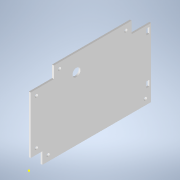
# Autodesk Inventor part: Steckerplatte_hint
Saved by Autodesk Inventor 2022 (Build 260153000, 153)
## iProperties
Created: 2022-02-01
Part Number: Steckerplatte_hint
Material: Generic
Document SubType Name: Modeling
Designer: Fabijansven
Density: 1 g/cm^3
Appearance: Default
Author: Fabijansven
Autodesk Inventor part; units mm, degrees
ref_plane "YZ Plane" through (0, 0, 0) normal (1, 0, 0) x (0, 1, 0)
ref_plane "XZ Plane" through (0, 0, 0) normal (0, 1, 0) x (-1, 0, 0)
ref_plane "XY Plane" through (0, 0, 0) normal (0, 0, 1) x (1, 0, 0)
sketch "Sketch1" plane through (0, 0, 0) normal (1, 0, 0) x (0, 1, 0)
  line L0 (0, 0) -> (140, 0)
  line L1 (140, 0) -> (140, -210)
  line L2 (140, -210) -> (0, -210)
  line L3 (0, -210) -> (0, 0)
  dimension "d0" = 210
  dimension "d1" = 140
  constraints: 8 end point, 2 parallel, 1 horizontal, 1 perpendicular
  measures "d0" distance of L0.end L1.end
  measures "d1" distance of L1.end L2.end
extrude "Extrusion1" add sketch "Sketch1" along normal blind 3
sketch "Sketch2" plane through (0, 0, 0) normal (-1, 0, 0) x (0, 0, 1)
  line L0 (0, 0) -> (-20.5, 0)
  line L1 (-20.5, 0) -> (-20.5, 20.5)
  line L2 (-20.5, 20.5) -> (0, 20.5)
  line L3 (0, 20.5) -> (0, 0)
  line L4 (-210, 140) -> (0, 140) projected
  line L5 (0, 140) -> (-40.5, 140)
  line L6 (-40.5, 140) -> (-40.5, 119.5)
  line L7 (-40.5, 119.5) -> (0, 119.5)
  line L8 (0, 119.5) -> (0, 140)
  line L9 (-210, 140) -> (-176, 140)
  line L10 (-176, 140) -> (-176, 119.5)
  line L11 (-176, 119.5) -> (-210, 119.5)
  line L12 (-210, 119.5) -> (-210, 140)
  point P0 (-176, 140)
  dimension "d4" = 20.5
  dimension "d5" = 20.5
  dimension "d6" = 40.5
  dimension "d7" = 20.5
  dimension "d8" = 34
  constraints: 24 end point, 6 parallel, 3 horizontal, 3 perpendicular, 1 point on line
  measures "d4" distance of L0.end L1.end
  measures "d5" distance of L5.end L6.end
  measures "d6" distance between parallel lines of L8 L6
  measures "d7" distance of L1.end L2.end
  measures "d8" distance between parallel lines of L12 L10
extrude "Extrusion2" cut sketch "Sketch2" against normal blind 3
sketch "Sketch3" plane through (0, 0, 0) normal (-1, 0, 0) x (0, 0, 1)
  circle A0 centre (-10, 30.5) radius 2.75
  line L0 (-20.5, 20.5) -> (0, 20.5) projected
  line L1 (0, 119.5) -> (0, 20.5) projected
  circle A1 centre (-10, 109.5) radius 2.75
  circle A2 centre (-50.5, 130) radius 2.75
  circle A3 centre (-166, 130) radius 2.75
  circle A4 centre (-200, 10) radius 2.75
  circle A5 centre (-30.5, 10) radius 2.75
  line L2 (-20.5, 0) -> (-210, 0) projected
  line L3 (-20.5, 0) -> (-20.5, 20.5) projected
  line L4 (-210, 0) -> (-210, 119.5) projected
  line L5 (-176, 140) -> (-176, 119.5) projected
  line L6 (-176, 140) -> (-40.5, 140) projected
  line L7 (-40.5, 119.5) -> (-40.5, 140) projected
  line L8 (0, 119.5) -> (-40.5, 119.5) projected
  point P0 (0, 0)
  dimension "d11" = 5.5
  dimension "d12" = 10
  dimension "d13" = 10
  dimension "d14" = 10
  dimension "d15" = 10
  dimension "d16" = 10
  dimension "d17" = 10
  dimension "d18" = 10
  dimension "d19" = 10
  dimension "d20" = 10
  dimension "d21" = 10
  dimension "d22" = 10
  dimension "d23" = 10
  dimension "d24" = 5.5
  dimension "d25" = 5.5
  dimension "d26" = 5.5
  dimension "d27" = 5.5
  dimension "d28" = 5.5
  constraints: 6 centre point
  measures "d11" diameter of A0
  measures "d12" distance from line of A0.centre L0
  measures "d13" distance from line of L1 A0.centre
  measures "d14" distance from line of L2 A5.centre
  measures "d15" distance from line of L3 A5.centre
  measures "d16" distance from line of L2 A4.centre
  measures "d17" distance from line of L4 A4.centre
  measures "d18" distance from line of L5 A3.centre
  measures "d19" distance from line of L6 A3.centre
  measures "d20" distance from line of L6 A2.centre
  measures "d21" distance from line of L7 A2.centre
  measures "d22" distance from line of L8 A1.centre
  measures "d23" distance from line of L1 A1.centre
  measures "d24" diameter of A1
  measures "d25" diameter of A5
  measures "d26" diameter of A4
  measures "d27" diameter of A3
  measures "d28" diameter of A2
extrude "Extrusion3" cut sketch "Sketch3" against normal blind 3
sketch "Sketch4" plane through (0, 0, 0) normal (-1, 0, 0) x (0, 0, 1)
  line L0 (-201.8, 25) -> (-207, 25)
  line L1 (-207, 25) -> (-207, 35.2)
  line L2 (-207, 35.2) -> (-201.8, 35.2)
  line L3 (-201.8, 35.2) -> (-201.8, 25)
  line L4 (-201.8, 104.8) -> (-207, 104.8)
  line L5 (-207, 104.8) -> (-207, 115)
  line L6 (-207, 115) -> (-201.8, 115)
  line L7 (-201.8, 115) -> (-201.8, 104.8)
  line L8 (-210, 0) -> (-210, 119.5) projected
  line L9 (-20.5, 0) -> (-210, 0) projected
  line L10 (-176, 119.5) -> (-210, 119.5) projected
  line L11 (-176, 140) -> (-40.5, 140) projected
  point P0 (0, 0)
  dimension "d31" = 3
  dimension "d32" = 25
  dimension "d34" = 10.2
  dimension "d35" = 10.2
  dimension "d36" = 5.2
  dimension "d37" = 25
  constraints: 16 end point, 4 parallel, 2 horizontal, 2 perpendicular, 2 point on line
  measures "d31" distance between parallel lines of L8 L1
  measures "d32" distance between parallel lines of L9 L0
  measures "d34" distance of L6.end L4.start
  measures "d35" distance of L2.end L0.start
  measures "d36" distance of L4.start L4.end
  measures "d37" distance between parallel lines of L6 L11
extrude "Extrusion4" cut sketch "Sketch4" against normal blind 3
sketch "Sketch5" plane through (0, 0, 0) normal (-1, 0, 0) x (0, 0, 1)
  point P0 (0, 0)
sketch "Sketch6" plane through (0, 0, 0) normal (-1, 0, 0) x (0, 0, 1)
  circle A0 centre (-80, 110) radius 7
  line L0 (-176, 140) -> (-40.5, 140) projected
  line L1 (0, 119.5) -> (0, 20.5) projected
  line L2 (-176, 140) -> (-176, 119.5) projected
  point P0 (0, 0)
  dimension "d40" = 14
  dimension "d41" = 30
  dimension "d43" = 80
  constraints: 1 centre point
  measures "d40" diameter of A0
  measures "d41" distance from line of A0.centre L0
  measures "d43" distance from line of A0.centre L1
extrude "Extrusion5" cut sketch "Sketch6" against normal blind 3
equation "\"d5\" = d4"
equation "\"d13\" = d12"
equation "\"d14\" = d12"
equation "\"d15\" = d12"
equation "\"d16\" = d12"
equation "\"d17\" = d12"
equation "\"d18\" = d12"
equation "\"d19\" = d12"
equation "\"d20\" = d12"
equation "\"d21\" = d12"
equation "\"d22\" = d12"
equation "\"d23\" = d12"
equation "\"d24\" = d11"
equation "\"d25\" = d11"
equation "\"d26\" = d11"
equation "\"d27\" = d11"
equation "\"d28\" = d11"
body "Solid1"
